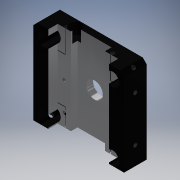
# Autodesk Inventor part: camera holder (G061008000)
Saved by Autodesk Inventor 2017 (Build 210142000, 142)
## iProperties
Part Number: camera holder (G061008000)
Material: Generisch
Document SubType Name: Modeling
Designer: David Merges
Density: 1 g/cm^3
Appearance: Eloxiert - schwarz
Author: David Merges
Autodesk Inventor part; units mm, degrees
note: some values were not read from the file. Chosen so that the rebuilt part matches the saved one: direction of "Bohrung4".
ref_plane "YZ Plane" through (0, 0, 0) normal (1, 0, 0) x (0, 1, 0)
ref_plane "XZ Plane" through (0, 0, 0) normal (0, 1, 0) x (-1, 0, 0)
ref_plane "XY Plane" through (0, 0, 0) normal (0, 0, 1) x (1, 0, 0)
sketch "Skizze1" plane through (0, 0, 0) normal (0, 1, 0) x (-1, 0, 0)
  line L0 (20, 20) -> (-20, 20)
  line L1 (-20, 20) -> (-20, -20)
  line L2 (-20, -20) -> (20, -20)
  line L3 (20, -20) -> (20, 20)
  line L4 (20, -20) -> (-20, 20) construction
  point P0 (0, 0)
  point P1 (0, 0)
  dimension "d0" = 40
  dimension "d1" = 40
  constraints: 10 end point, 2 parallel, 1 coincident, 1 horizontal, 1 midpoint, 1 perpendicular
  measures "d0" distance of L2.end L1.end
  measures "d1" distance of L1.end L0.end
extrude "Extrusion1" add sketch "Skizze1" along normal mid plane 10
sketch "Skizze2" plane through (0, -5, 0) normal (0, -1, 0) x (1, 0, 0)
  line L0 (-15, 15) -> (15, 15) construction
  line L1 (15, 15) -> (15, -15) construction
  line L2 (15, -15) -> (-15, -15) construction
  line L3 (-15, -15) -> (-15, 15) construction
  line L4 (15, -15) -> (-15, 15) construction
  point P0 (0, 0)
  dimension "d4" = 30
  dimension "d5" = 30
  constraints: 10 end point, 2 midpoint, 2 parallel, 1 horizontal, 1 perpendicular
  measures "d4" distance of L1.end L2.end
  measures "d5" distance of L0.end L1.end
hole "Bohrung1" at (15, -5, -15) at (15, -5, 15) at (-15, -5, 15) at (-15, -5, -15) direction (0, 1, 0) diameter 6 end through all
sketch "Skizze3" plane through (0, -5, 0) normal (0, -1, 0) x (1, 0, 0)
  circle A0 centre (-15, 15) radius 3 projected
  circle A1 centre (15, -15) radius 3 projected
  circle A2 centre (15, 15) radius 3 projected
  circle A3 centre (-15, -15) radius 3 projected
  line L0 (20, 20) -> (-20, 20) projected
  line L1 (-20, 20) -> (-20, -20) projected
  line L2 (-20, -20) -> (20, -20) projected
  line L3 (20, -20) -> (20, 20) projected
  line L4 (-20, 18.2322) -> (-18.2322, 20)
  line L5 (-20, 20) -> (20, 20) projected
  line L6 (20, 20) -> (-20, 20) projected
  line L7 (-18.2322, 20) -> (-20, 20)
  line L8 (-20, 20) -> (-20, 18.2322)
  point P0 (0, 0)
  dimension "d13" = 45
  dimension "d14" = 2.5
  constraints: 6 end point, 2 collinear, 2 point on line
  measures "d13" angle of L0 L4
  measures "d14" distance of L4.start L4.end
extrude "Extrusion2" cut sketch "Skizze3" against normal through all contours L4 L1 L0
pattern_circular "Runde Anordnung1" count 4 over 360 about axis through (0, -10, 0) along (0, 1, 0) of "Extrusion2"
sketch "Skizze4" plane through (0, -5, 0) normal (0, -1, 0) x (1, 0, 0)
  circle A0 centre (0, 0) radius 3.65
  dimension "d20" = 7.3
  constraints: 1 centre point, 1 coincident
  measures "d20" diameter of A0
extrude "Extrusion3" cut sketch "Skizze4" against normal through all
sketch "Skizze5" plane through (0, -5, 0) normal (0, -1, 0) x (1, 0, 0)
  circle A0 centre (0, 0) radius 3.65 projected
  line L0 (-20, -18.2322) -> (-18.2322, -20) projected
  line L1 (-18.2322, -20) -> (18.2322, -20) projected
  line L2 (18.2322, -20) -> (20, -18.2322) projected
  line L3 (20, -18.2322) -> (20, 18.2322) projected
  line L4 (20, 18.2322) -> (18.2322, 20) projected
  line L5 (18.2322, 20) -> (-18.2322, 20) projected
  line L6 (-18.2322, 20) -> (-20, 18.2322) projected
  line L7 (-20, 18.2322) -> (-20, -18.2322) projected
  circle A1 centre (-15, 15) radius 3 projected
  circle A2 centre (15, -15) radius 3 projected
  circle A3 centre (15, 15) radius 3 projected
  circle A4 centre (-15, -15) radius 3 projected
  line L8 (-18.2322, 20) -> (18.2322, 20) projected
  line L9 (18.2322, -20) -> (-18.2322, -20) projected
  line L10 (-7.5, 20) -> (7.5, 20)
  line L11 (7.5, 20) -> (7.5, -20)
  line L12 (7.5, -20) -> (-7.5, -20)
  line L13 (-7.5, -20) -> (-7.5, 20)
  line L14 (7.5, -20) -> (-7.5, 20) construction
  dimension "d23" = 15
  constraints: 10 end point, 2 parallel, 2 point on line, 1 coincident, 1 horizontal, 1 midpoint, 1 perpendicular
  measures "d23" distance between parallel lines of L13 L11
extrude "Extrusion4" cut sketch "Skizze5" against normal blind 7 contours L13 L5 L11 L1
sketch "Skizze6" plane through (0, -5, 0) normal (0, -1, 0) x (1, 0, 0)
  circle A0 centre (-15, -15) radius 3 projected
  circle A1 centre (-15, 15) radius 3 projected
  line L0 (-7.5, -20) -> (-7.5, 20) projected
  line L1 (-7.5, 20) -> (-18.2322, 20) projected
  line L2 (-18.2322, 20) -> (-20, 18.2322) projected
  line L3 (-20, 18.2322) -> (-20, -18.2322) projected
  line L4 (-20, -18.2322) -> (-18.2322, -20) projected
  line L5 (-18.2322, -20) -> (-7.5, -20) projected
  line L6 (7.5, 20) -> (7.5, -20) projected
  line L7 (7.5, -20) -> (18.2322, -20) projected
  line L8 (18.2322, -20) -> (20, -18.2322) projected
  line L9 (20, -18.2322) -> (20, 18.2322) projected
  line L10 (20, 18.2322) -> (18.2322, 20) projected
  line L11 (18.2322, 20) -> (7.5, 20) projected
  circle A2 centre (15, -15) radius 3 projected
  circle A3 centre (15, 15) radius 3 projected
  line L12 (-7.5, 20) -> (-18.2322, 20) projected
  line L13 (18.2322, -20) -> (-18.2322, -20) projected
  line L14 (-13.3, 20) -> (13.3, 20)
  line L15 (13.3, 20) -> (13.3, -20)
  line L16 (13.3, -20) -> (-13.3, -20)
  line L17 (-13.3, -20) -> (-13.3, 20)
  line L18 (13.3, -20) -> (-13.3, 20) construction
  point P0 (0, 0)
  point P1 (0, 0)
  dimension "d26" = 26.6
  constraints: 10 end point, 2 parallel, 2 point on line, 1 coincident, 1 horizontal, 1 midpoint, 1 perpendicular
  measures "d26" distance between parallel lines of L15 L17
extrude "Extrusion5" cut sketch "Skizze6" against normal blind 4.1 contours A0 L17 | A0 L17 A1 L1 L0 L5 | L17 A1 | L0 L14 L6 L13 | L6 L11 L15 A3 A2 L7 | A2 L15 | L15 A3 picked at (-13.119, -14.3359) picked at (-12.7148, 14.6004) picked at (12.5047, -15) picked at (12.8667, 15)
sketch "Skizze7" plane through (0, -0.9, 0) normal (0, -1, 0) x (1, 0, 0)
  circle A0 centre (-10.4, -12.5) radius 1.1 projected
  circle A1 centre (-10.4, 0) radius 1.1 projected
  circle A2 centre (10.4, 0) radius 1.1 projected
  circle A3 centre (10.4, -12.5) radius 1.1 projected
  point P0 (0, 0)
hole "Bohrung2" at (10.4, -0.9, -12.5) at (10.4, -0.9, 0) at (-10.4, -0.9, -12.5) at (-10.4, -0.9, 0) direction (0, 1, 0) diameter 1.567 end through all thread size "M2x0.4" class "6H" standard "ISO Metric profile"
sketch "Skizze8" plane through (20, -5, -18.2322) normal (1, 0, 0) x (0, 0, -1)
  line L0 (-36.4645, 10) -> (-36.4645, 0) projected
  line L1 (0, 0) -> (0, 10) projected
  line L2 (-28.2322, 5) -> (-8.2322, 5) construction
  line L3 (-36.4645, 0) -> (-36.4645, 10) construction
  line L4 (-36.4645, 0) -> (0, 10) construction
  point P0 (-18.2322, 5)
  dimension "d37" = 20
  constraints: 4 end point, 2 coincident, 2 midpoint, 1 perpendicular
  measures "d37" distance of L2.start L2.end
hole "Bohrung3" at (20, 0, 10) at (20, 0, -10) direction (-1, 0, 0) diameter 1.813 depth 10 tip angle 118 thread size "M2.3x0.45" class "6H" standard "ISO Metric profile"
pattern_circular "Runde Anordnung2" count 4 over 360 about axis through (0, -10, 0) along (0, 1, 0) of "Bohrung3"
sketch "Skizze9" plane through (18.2322, -5, 20) normal (0.7071068, 0, 0.7071068) x (0.7071068, 0, -0.7071068)
  line L0 (2.5, 0) -> (0, 0) projected
  line L1 (0, 10) -> (2.5, 10) projected
  line L2 (2.5, 10) -> (2.5, 0) construction
  line L3 (0, 10) -> (0, 0) construction
  line L4 (2.5, 0) -> (0, 10) construction
  point P0 (1.25, 5)
  point P1 (1.25, 5)
  constraints: 2 end point, 1 coincident
hole "Bohrung4" at (19.1161, 0, 19.1161) direction (-0.7071068, 0, -0.7071068) diameter 1.813 end up to surface thread size "M2.3x0.45" class "6H" standard "ISO Metric profile"
pattern_circular "Runde Anordnung3" count 4 over 360 about axis through (0, -10, 0) along (0, 1, 0) of "Bohrung4"
sketch "Skizze10" plane through (-18.2322, -5, 20) normal (0, 0, 1) x (1, 0, 0)
  arc A0 (8.3406, 4.1) -> (8.1239, 4.1) centre (8.2322, 5) ccw projected
  line L0 (8.3406, 4.1) -> (10.7322, 4.1) projected
  line L1 (10.7322, 4.1) -> (10.7322, 7) projected
  line L2 (10.7322, 7) -> (25.7322, 7) projected
  line L3 (25.7322, 7) -> (25.7322, 4.1) projected
  line L4 (25.7322, 4.1) -> (28.1239, 4.1) projected
  arc A1 (28.3406, 4.1) -> (28.1239, 4.1) centre (28.2322, 5) ccw projected
  line L5 (28.3406, 4.1) -> (31.5322, 4.1) projected
  line L6 (31.5322, 4.1) -> (31.5322, 0) projected
  line L7 (36.4645, 0) -> (31.5322, 0) projected
  line L8 (36.4645, 0) -> (36.4645, 10) projected
  line L9 (0, 10) -> (36.4645, 10) projected
  line L10 (0, 10) -> (0, 0) projected
  line L11 (4.9322, 0) -> (0, 0) projected
  line L12 (4.9322, 0) -> (4.9322, 4.1) projected
  line L13 (4.9322, 4.1) -> (8.1239, 4.1) projected
  line L14 (10.7322, 4.1) -> (10.7322, 7) construction
  point P0 (18.2322, 5)
  point P1 (9.7322, 7.05)
  dimension "d59" = 2.95
  dimension "d60" = 5.9
  dimension "d61" = 1
  measures "d59" distance from line of L13 point (9.732, 7.05)
  measures "d60" distance between parallel lines of L9 L13
  measures "d61" distance from line of point (9.732, 7.05) L1
hole "Bohrung5" at (-8.5, 2.05, 20) direction (0, 0, -1) diameter 5 depth 5
sketch "Skizze11" plane through (18.2322, 5, -20) normal (0, 0, -1) x (-1, 0, 0)
  line L0 (-25.6195, 25.3163) -> (54.0474, 25.3163)
  line L1 (54.0474, 25.3163) -> (54.0474, -51.3074)
  line L2 (54.0474, -51.3074) -> (-25.6195, -51.3074)
  line L3 (-25.6195, -51.3074) -> (-25.6195, 25.3163)
  point P0 (18.2322, -5)
  constraints: 8 end point, 2 parallel, 1 horizontal, 1 perpendicular
extrude "Extrusion6" cut sketch "Skizze11" against normal blind 2
equation "\"d59\" = 0.5 * d60"
